Atap Single Slope (Autodesk Fusion 360 archive; units mm, degrees)
design "Solar Collector Fluida Udara"
part number: 2025-10-13-20-22-01-862
Autodesk Fusion 360 part; units mm, degrees
sketch "Sketch1" plane through (0, 0, 0) normal (0, 1, 0) x (1, 0, 0)
  line L0 (75, 300) -> (-75, 300)
  line L1 (-75, 300) -> (-75, -300)
  line L2 (-75, -300) -> (75, -300)
  line L3 (75, -300) -> (75, 300)
  line L4 (75, 300) -> (-75, -300) construction
  line L5 (-75, 300) -> (75, -300) construction
  dimension "d1" = 150
  dimension "d2" = 600
  constraint horizontal L0
  constraint perpendicular L0 L1
  constraint parallel L0 L2
  constraint parallel L1 L3
  constraint coincident L4 origin
  constraint coincident L5 origin
  measures "d1" distance of L1.end L2.end
  measures "d2" distance of L0.end L1.end
extrude "Extrude1" add sketch "Sketch1" along normal blind 900 makes body 1
move_body "Move1" bodies 1 to x (0.173648, -0.984808, 0) y (0.984808, 0.173648, 0) z (0, 0, 1) at (-61.9764, -73.8606, 0)
ref_plane "WorkPlane1" through (-61.9764, -73.8606, 0) normal (-0.984808, -0.173648, 0) x (-0.173648, 0.984808, 0)
sketch "Sketch2" plane through (-72.7385, -12.8258, 0) normal (-0.984808, -0.173648, 0) x (-0.173648, 0.984808, 0)
  circle A0 centre (-50, 250) radius 25
  circle A1 centre (-53.0509, 150) radius 25
  circle A2 centre (-53.0509, 49.9919) radius 25
  circle A3 centre (-53.0509, -49.1143) radius 25
  dimension "d7" = 50
  dimension "d8" = 50
  dimension "d9" = 50
  dimension "d10" = 50
  measures "d7" diameter of A0
  measures "d8" diameter of A1
  measures "d9" diameter of A2
  measures "d10" diameter of A3
shell "Shell1" thickness 10 removed faces 0 bodies 1
extrude "Extrude2" cut sketch "Sketch2" against normal blind 10 bodies 1
ref_plane "WorkPlane2" through (824.3506, 82.4228, 0) normal (0.984808, 0.173648, 0) x (0, 0, 1)
sketch "Sketch3" plane through (813.5885, 143.4576, 0) normal (0.984808, 0.173648, 0) x (0, 0, 1)
  line L0 (285, 125) -> (-285, 125)
  line L1 (-285, 125) -> (-285, -5)
  line L2 (-285, -5) -> (285, -5)
  line L3 (285, -5) -> (285, 125)
  line L4 (285, 125) -> (-285, -5) construction
  line L5 (-285, 125) -> (285, -5) construction
  point P0 (0, 60)
  dimension "d15" = 570
  dimension "d16" = 130
  constraint horizontal L0
  constraint perpendicular L0 L1
  constraint parallel L0 L2
  constraint parallel L1 L3
  constraint coincident L4 P0
  constraint coincident L5 P0
  measures "d15" distance of L1.end L2.end
  measures "d16" distance of L0.end L1.end
extrude "Extrude3" cut sketch "Sketch3" against normal blind 850 bodies 1
ref_plane "WorkPlane3" through (-61.9764, -73.8606, 0) normal (-0.984808, -0.173648, 0) x (-0.173648, 0.984808, 0)
sketch "Sketch4" plane through (-72.7385, -12.8258, 0) normal (-0.984808, -0.173648, 0) x (-0.173648, 0.984808, 0)
  circle A0 centre (-50, -150) radius 25
  circle A1 centre (-50, -250) radius 25
  dimension "d20" = 50
  dimension "d21" = 50
  measures "d20" diameter of A0
  measures "d21" diameter of A1
extrude "Extrude4" cut sketch "Sketch4" against normal blind 10 bodies 1
ref_plane "WorkPlane4" through (824.3506, 82.4228, 0) normal (0.984808, 0.173648, 0) x (0, 0, 1)
sketch "Sketch5" plane through (813.5885, 143.4576, 0) normal (0.984808, 0.173648, 0) x (0, 0, 1)
  line L0 (-300, -13) -> (300, -13)
  line L1 (300, -13) -> (300, 137)
  line L2 (300, 137) -> (-300, 137)
  line L3 (-300, 137) -> (-300, -13)
  dimension "d25" = 600
  dimension "d26" = 150
  constraint horizontal L0
  constraint vertical L1
  constraint horizontal L2
  constraint vertical L3
  measures "d25" distance of L0.start L0.end
  measures "d26" distance of L0.start L2.end
extrude "Extrude5" cut sketch "Sketch5" against normal blind 100 bodies 1
delete_face "DeleteFace1" 1 faces at (778.5042, 150.4718, -100) on bodies 1
ref_plane "WorkPlane5" through (-61.9764, -73.8606, 0) normal (-0.984808, -0.173648, 0) x (-0.173648, 0.984808, 0)
sketch "Sketch6" plane through (-72.7385, -12.8258, 0) normal (-0.984808, -0.173648, 0) x (-0.173648, 0.984808, 0)
  line L0 (-136.9764, -300) -> (13.0236, -300)
  line L1 (13.0236, -300) -> (13.0236, 300)
  line L2 (13.0236, 300) -> (-136.9764, 300)
  line L3 (-136.9764, 300) -> (-136.9764, -300)
  line L4 (4.4986, 290) -> (-125.5014, 290)
  line L5 (-125.5014, 290) -> (-125.5014, -290)
  line L6 (-125.5014, -290) -> (4.4986, -290)
  line L7 (4.4986, -290) -> (4.4986, 290)
  line L8 (4.4986, 290) -> (-125.5014, -290) construction
  line L9 (-125.5014, 290) -> (4.4986, -290) construction
  point P0 (-136.9764, -300)
  point P1 (13.0236, 300)
  point P2 (-60.5014, 0)
  dimension "d30" = 130
  dimension "d31" = 580
  constraint horizontal L0
  constraint vertical L1
  constraint horizontal L2
  constraint vertical L3
  constraint coincident P1 L1.end
  constraint coincident P0 L0.start
  constraint horizontal L4
  constraint perpendicular L4 L5
  constraint parallel L4 L6
  constraint parallel L5 L7
  constraint coincident L8 P2
  constraint coincident L9 P2
  measures "d30" distance of L5.end L6.end
  measures "d31" distance of L4.end L5.end
extrude "Extrude6" add sketch "Sketch6" along normal blind 100 separate body makes body 2
ref_plane "WorkPlane6" through (-98.1932, -156.4036, 0) normal (0.173648, -0.984808, 0) x (0, 0, 1)
